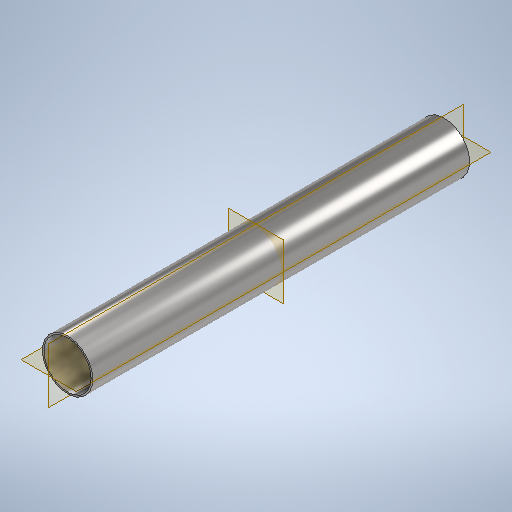
# Autodesk Inventor part: Sessao_28_03_002_001
Saved by Autodesk Inventor 2026 (Build 300175000, 175)
## iProperties
Created: 2025-03-28
Part Number: Sessao_28_03_002_001
Material: Steel, Galvanized
Document SubType Name: Sheet Metal
Designer: Carlos Dias
Density: 7.85 g/cm^3
Sheet Metal Rule: Default
Appearance: Galvanized
Author: Carlos Dias
Autodesk Inventor part; units mm, degrees
sketch "Sketch2" plane through (0, 0, 0) normal (0, 0, 1) x (1, 0, 0)
  circle A0 centre (0, 0) radius 50
  circle A1 centre (0, 0) radius 47
  dimension "d5" = 100
  dimension "d6" = 3
  constraints: 2 centre point, 2 coincident
  measures "d5" diameter of A0
  measures "d6" radial gap between concentric circles of A0 A1
extrude "Extrusion2" add sketch "Sketch2" along normal mid plane 750
equation "\"BendRadius\" = Thickness"
equation "\"BendReliefWidth\" = Thickness"
equation "\"BendReliefDepth\" = 0.5 * Thickness"
equation "\"CornerReliefSize\" = 4 * Thickness"
equation "\"MinimumRemnant\" = 2 * Thickness"
equation "\"TransitionRadius\" = BendRadius"
equation "\"JacobiRadiusSize\" = BendRadius"
equation "\"GapSize\" = Thickness"
equation "\"Thickness\" = 3.048"
body "Solid2"
